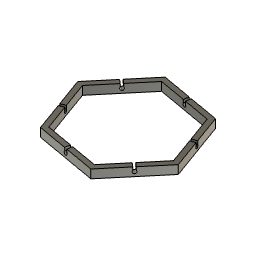
ServoBase2 v2 (Autodesk Fusion 360 design; units mm, degrees)
Autodesk Fusion 360 part; units mm, degrees
sketch "Sketch1" plane through (0, 0, 0) normal (0, 0, 1) x (1, 0, 0)
  line L0 (-10.798, 13.3938) -> (-13.526, 20.8958)
  line L1 (-9.4934, 25.6987) -> (-13.526, 20.8958)
  line L2 (19.2845, 47.1681) -> (9.9209, 48.822)
  line L3 (55.6112, 15.5789) -> (58.2905, 8.2107)
  line L4 (52.0708, 0.8027) -> (58.2905, 8.2107)
  line L5 (8.3931, -15.0435) -> (-1.0646, -13.373)
  line L6 (-10.798, 13.3938) -> (-9.5166, 9.87)
  line L7 (-5.074, -2.3473) -> (-1.0646, -13.373)
  line L8 (1.1628, -10.72) -> (-2.2546, -1.322)
  line L9 (-6.6972, 10.8953) -> (-10.1147, 20.2932)
  line L10 (33.6598, -16.4599) -> (23.8122, -14.7206)
  line L11 (11.0104, -12.4594) -> (1.1628, -10.72)
  line L12 (8.3931, -15.0435) -> (10.4886, -15.4136)
  line L13 (23.2904, -17.6748) -> (34.8436, -19.7155)
  line L14 (54.8793, 8.8133) -> (48.4491, 1.1547)
  line L15 (40.0899, -8.8014) -> (33.6598, -16.4599)
  line L16 (52.0708, 0.8027) -> (50.7467, -0.7743)
  line L17 (42.3875, -10.7304) -> (34.8436, -19.7155)
  line L18 (43.6017, 39.8265) -> (47.0192, 30.4285)
  line L19 (51.4618, 18.2112) -> (54.8793, 8.8133)
  line L20 (55.6112, 15.5789) -> (54.2812, 19.2364)
  line L21 (49.8385, 31.4537) -> (45.8292, 42.4795)
  line L22 (11.1048, 45.5664) -> (20.9523, 43.827)
  line L23 (33.7542, 41.5658) -> (43.6017, 39.8265)
  line L24 (19.2845, 47.1681) -> (21.4741, 46.7813)
  line L25 (34.276, 44.5201) -> (45.8292, 42.4795)
  line L26 (-10.1147, 20.2932) -> (-3.6845, 27.9518)
  line L27 (4.6746, 37.9079) -> (11.1048, 45.5664)
  line L28 (-9.4934, 25.6987) -> (-5.9821, 29.8808)
  line L29 (2.3771, 39.8369) -> (9.9209, 48.822)
  line L30 (50.7467, -0.7743) -> (42.3875, -10.7304)
  line L31 (40.0899, -8.8014) -> (48.4491, 1.1547)
  line L32 (23.2904, -17.6748) -> (10.4886, -15.4136)
  line L33 (11.0104, -12.4594) -> (23.8122, -14.7206)
  line L34 (-2.2546, -1.322) -> (-6.6972, 10.8953)
  line L35 (-9.5166, 9.87) -> (-5.074, -2.3473)
  line L36 (-3.6845, 27.9518) -> (4.6746, 37.9079)
  line L37 (2.3771, 39.8369) -> (-5.9821, 29.8808)
  line L38 (20.9523, 43.827) -> (33.7542, 41.5658)
  line L39 (34.276, 44.5201) -> (21.4741, 46.7813)
  line L40 (49.8385, 31.4537) -> (54.2812, 19.2364)
  line L41 (51.4618, 18.2112) -> (47.0192, 30.4285)
  constraint coincident L7.start L6
  constraint collinear L6 L7
  constraint collinear L8 L9
  constraint coincident L25.start L24
  constraint coincident L29.start L28
  constraint coincident L13.start L12
  constraint coincident L17.start L16
  constraint coincident L21.start L20
  constraint collinear L10 L11
  constraint collinear L12 L13
  constraint collinear L14 L15
  constraint collinear L16 L17
  constraint collinear L18 L19
  constraint collinear L20 L21
  constraint collinear L22 L23
  constraint collinear L24 L25
  constraint collinear L26 L27
  constraint collinear L28 L29
  constraint parallel L30 L31
  constraint parallel L32 L33
  constraint parallel L34 L35
  constraint parallel L36 L37
  constraint parallel L38 L39
  constraint parallel L40 L41
extrude "Extrude1" add sketch "Sketch1" along normal blind 5
sketch "Sketch2" plane through (8.6627, 49.0442, 0) normal (0.173939, 0.984757, 0) x (-0.984757, 0.173939, 0)
  line L0 (-37.7418, 0) -> (-1.2777, 0)
  line L1 (-1.2777, 0) -> (-1.2777, 5)
  line L2 (-1.2777, 5) -> (-37.7418, 5)
  line L3 (-37.7418, 5) -> (-37.7418, 0)
  line L4 (-20.2597, 5) -> (-20.2597, 3.1614)
  line L5 (-18.7597, 3.1614) -> (-18.7597, 5)
  arc A0 (-20.2597, 3.1614) -> (-18.7597, 3.1614) centre (-19.5097, 2.5) ccw
  arc A1 (-19.3816, 3.4918) -> (-19.5097, 3.5) centre (-19.5097, 2.5) ccw
  line L6 (-20.2597, 5) -> (-18.7597, 5)
  arc A2 (-20.2597, 3.1614) -> (-18.7597, 3.1614) centre (-19.5097, 2.5) ccw
  line L7 (-18.7597, 3.1614) -> (-18.7597, 5)
  line L8 (-20.2597, 5) -> (-20.2597, 3.1614)
  line L9 (-20.2597, 5) -> (-18.7597, 5)
  arc A3 (-20.2597, 3.1614) -> (-18.7597, 3.1614) centre (-19.5097, 2.5) ccw
  line L10 (-18.7597, 3.1614) -> (-18.7597, 5)
  line L11 (-20.2597, 5) -> (-20.2597, 3.1614)
  line L12 (-20.2597, 5) -> (-18.7597, 5)
  point P0 (-19.5097, 2.5)
  dimension "d30" = 2
  dimension "d34" = 2
  dimension "d35" = 2
  constraint coincident P0 A0.centre
  constraint coincident L2 L5.end
  constraint coincident L2 L4.start
  constraint coincident A1.start A0
  constraint concentric A0 A1
  constraint perpendicular L5 L6
  constraint perpendicular L7 L9
  constraint perpendicular L10 L12
  measures "d30" diameter of A0
  measures "d34" diameter of A2
  measures "d35" diameter of A3
sketch "Sketch3" plane through (-18.2237, 15.3006, 0) normal (-0.765855, 0.643013, 0) x (-0.643013, -0.765855, 0)
  line L0 (-43.7698, 0) -> (-7.3057, 0)
  line L1 (-7.3057, 0) -> (-7.3057, 5)
  line L2 (-7.3057, 5) -> (-43.7698, 5)
  line L3 (-43.7698, 5) -> (-43.7698, 0)
  arc A0 (-26.2597, 3.1614) -> (-24.7597, 3.1614) centre (-25.5097, 2.5) ccw
  line L4 (-24.7597, 3.1614) -> (-24.7597, 5)
  line L5 (-26.2597, 5) -> (-26.2597, 3.1614)
  line L6 (-26.2597, 5) -> (-24.7597, 5)
  dimension "d36" = 2
  constraint perpendicular L4 L6
  measures "d36" diameter of A0
sketch "Sketch4" plane through (-5.2353, -1.9037, 0) normal (-0.939793, -0.341743, 0) x (0.341743, -0.939793, 0)
  line L0 (-24.2601, 0) -> (12.204, 0)
  line L1 (12.204, 0) -> (12.204, 5)
  line L2 (12.204, 5) -> (-24.2601, 5)
  line L3 (-24.2601, 5) -> (-24.2601, 0)
  arc A0 (-6.7597, 3.1614) -> (-5.2597, 3.1614) centre (-6.0097, 2.5) ccw
  line L4 (-5.2597, 3.1614) -> (-5.2597, 5)
  line L5 (-6.7597, 5) -> (-6.7597, 3.1614)
  line L6 (-6.7597, 5) -> (-5.2597, 5)
  dimension "d39" = 2
  constraint perpendicular L4 L6
  measures "d39" diameter of A0
extrude "Extrude5" cut sketch "Sketch2" against normal blind 69 contours L2 L4 L5 A0 L6 A2 L7 L8 L9 A3 L10 L11 L12
extrude "Extrude6" cut sketch "Sketch3" against normal blind 67 contours L2 A0 L4 L5 L6
extrude "Extrude7" cut sketch "Sketch4" against normal blind 67 contours L2 A0 L4 L5 L6
